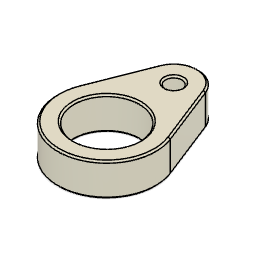
bottom slider v2 (Autodesk Fusion 360 design; units mm, degrees)
Autodesk Fusion 360 part; units mm, degrees
sketch "Sketch1" plane through (0, 0, 0) normal (0, 1, 0) x (1, 0, 0)
  circle A0 centre (0, 0) radius 20
  line L0 (-13.9601, 46.4878) -> (-27.9202, 10.9756)
  arc A1 (-27.9202, 10.9756) -> (27.9202, 10.9756) centre (0, 0) ccw
  line L1 (27.9202, 10.9756) -> (13.9601, 46.4878)
  arc A2 (13.9601, 46.4878) -> (-13.9601, 46.4878) centre (0, 41) ccw
  circle A3 centre (0, 41) radius 5
  point P0 (0, -30)
  point P1 (0, 56)
  dimension "d1" = 40
  dimension "d2" = 30
  dimension "d3" = 41
  dimension "d4" = 15
  dimension "d8" = 10
  dimension "d9" = 86
  constraint coincident A0.centre A1.centre
  constraint tangent L0 A1
  constraint tangent A1 L1
  constraint tangent L1 A2
  constraint tangent L0 A2
  constraint vertical A0.centre A2.centre
  constraint concentric A2 A3
  constraint midpoint A1 P0
  constraint midpoint A2 P1
  measures "d1" diameter of A0
  measures "d2" radius of A1
  measures "d3" vertical distance of A0.centre A2.centre
  measures "d4" radius of A2
  measures "d8" diameter of A3
  measures "d9" distance of P0 P1
extrude "Extrude1" add sketch "Sketch1" along normal blind 20
chamfer "Chamfer1" distance 1 angle 45 12 edges at (0, 20, -56) (-20.9401, 20, -28.7317) (0, 20, 30) (20.9401, 20, -28.7317) (0, 0, -56) (-20.9401, 0, -28.7317) (0, 0, 30) (20.9401, 0, -28.7317) (-18.6465, 20, -7.2323) (-18.6465, 0, -7.2323) (-4.6616, 20, -42.8081) (-4.6616, 0, -42.8081)
